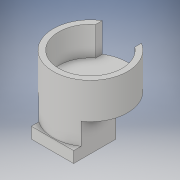
# Autodesk Inventor part: stepper_housing
Saved by Autodesk Inventor 2017 (Build 210142000, 142)
## iProperties
Created: 2017-01-20
Part Number: stepper_housing
Material: Generic
Document SubType Name: Modeling
Designer: Gabe Madonna
Density: 1 g/cm^3
Appearance: Default
Author: Gabe Madonna
Autodesk Inventor part; units mm, degrees
ref_plane "YZ Plane" through (0, 0, 0) normal (1, 0, 0) x (0, 1, 0)
ref_plane "XZ Plane" through (0, 0, 0) normal (0, 1, 0) x (-1, 0, 0)
ref_plane "XY Plane" through (0, 0, 0) normal (0, 0, 1) x (1, 0, 0)
sketch "Sketch1" plane through (0, 0, 0) normal (0, 1, 0) x (-1, 0, 0)
  circle A0 centre (0, 0) radius 14.15
  circle A1 centre (0, 0) radius 16.574
  dimension "d0" = 28.3
  dimension "d1" = 2.424
  constraints: 2 centre point, 1 coincident
  measures "d0" diameter of A0
  measures "d1" radial gap between concentric circles of A0 A1
extrude "Extrusion1" add sketch "Sketch1" along normal blind 13
sketch "Sketch2" plane through (0, 0, 0) normal (0, -1, 0) x (1, 0, 0)
  circle A0 centre (0, 0) radius 16.574 projected
extrude "Extrusion2" add sketch "Sketch2" along normal blind 3
sketch "Sketch3" plane through (0, 13, 0) normal (0, 1, 0) x (1, 0, 0)
  line L0 (0, 16.574) -> (-8.75, 16.574)
  line L1 (-8.75, 16.574) -> (8.75, 16.574)
  line L2 (-8.75, 16.574) -> (8.75, 16.574)
  line L3 (8.75, 16.574) -> (8.75, 5.314)
  line L4 (8.75, 5.314) -> (-8.75, 5.314)
  line L5 (-8.75, 5.314) -> (-8.75, 16.574)
  dimension "d6" = 8.75
  dimension "d7" = 17.5
  constraints: 12 end point, 2 horizontal, 2 parallel, 1 perpendicular, 1 point on line
  measures "d6" distance of L0.start L0.end
  measures "d7" distance of L0.end L1.end
extrude "Extrusion3" cut sketch "Sketch3" against normal up to surface (13 mm away)
sketch "Sketch4" plane through (0, -3, 0) normal (0, -1, 0) x (1, 0, 0)
  arc A0 (8.75, -14.076) -> (-8.75, -14.076) centre (0, 0) ccw projected
  line L0 (0, 16.574) -> (0, 2.9438)
  line L1 (0, 2.9438) -> (0, 12.0338)
  line L2 (-9.45, -1.9612) -> (-9.45, 16.9388)
  line L3 (-9.45, 16.9388) -> (9.45, 16.9388)
  line L4 (9.45, 16.9388) -> (9.45, -1.9612)
  line L5 (9.45, -1.9612) -> (-9.45, -1.9612)
  point P0 (0.0791, 7.4888)
  point P1 (0, 7.4888)
  point P2 (0, -1.9612)
  dimension "d13" = 18.9
  constraints: 12 end point, 2 midpoint, 2 point on line, 1 point on circle, 1 vertical, 9 other
  measures "d13" distance of L3.end L4.end
extrude "Extrusion4" add sketch "Sketch4" along normal blind 14.7
sketch "Sketch5" plane through (0, -3, 0) normal (0, 1, 0) x (1, 0, 0)
  arc A0 (-9.45, -13.616) -> (9.45, -13.616) centre (0, 0) ccw projected
  line L0 (-9.45, -13.616) -> (-9.45, -16.9388) projected
  line L1 (-9.45, -16.9388) -> (9.45, -16.9388) projected
  line L2 (9.45, -16.9388) -> (9.45, -13.616) projected
extrude "Extrusion5" cut sketch "Sketch5" against normal blind 9.7
body "Solid1"
